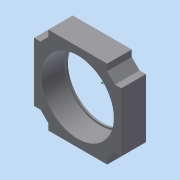
# Autodesk Inventor part: 20_Lens_holder_DIA_50mm
Saved by Autodesk Inventor 2019.4 (Build 234330000, 330)
## iProperties
Created: 2019-10-23
Part Number: 20_Lens_holder_DIA_50mm
Material: Generic
Document SubType Name: Modeling
Designer: marsikovabarbora
Density: 1 g/cm^3
Appearance: Default
Lens_diameter: 25,400 mm
Author: marsikovabarbora
Autodesk Inventor part; units mm, degrees
ref_plane "YZ Plane" through (0, 0, 0) normal (1, 0, 0) x (0, 1, 0)
ref_plane "XZ Plane" through (0, 0, 0) normal (0, 1, 0) x (-1, 0, 0)
ref_plane "XY Plane" through (0, 0, 0) normal (0, 0, 1) x (1, 0, 0)
sketch "Sketch1" plane through (0, 0, 0) normal (0, 0, 1) x (1, 0, 0)
  line L0 (-34.8609, 0) -> (34.8609, 0) construction
  line L1 (0, -34.8609) -> (0, 34.8609) construction
  line L2 (0, 0) -> (13.4339, 13.4339) construction
  line L3 (0, 0) -> (18.9985, 0) construction
  line L4 (0, 24.9006) -> (16.8, 24.9006)
  line L5 (16.8, 24.9006) -> (16.8, 21.2406)
  line L6 (16.8, 21.2406) -> (19.0203, 19.0203)
  line L7 (24.9006, 0) -> (24.9006, 16.8)
  line L8 (24.9006, 16.8) -> (21.2406, 16.8)
  line L9 (21.2406, 16.8) -> (19.0203, 19.0203)
  line L10 (0, 0) -> (-13.4339, 13.4339) construction
  line L11 (0, 0) -> (-18.9985, 0) construction
  line L12 (0, 24.9006) -> (-16.8, 24.9006)
  line L13 (-16.8, 24.9006) -> (-16.8, 21.2406)
  line L14 (-16.8, 21.2406) -> (-19.0203, 19.0203)
  line L15 (-24.9006, 0) -> (-24.9006, 16.8)
  line L16 (-24.9006, 16.8) -> (-21.2406, 16.8)
  line L17 (-21.2406, 16.8) -> (-19.0203, 19.0203)
  line L18 (0, 0) -> (13.4339, -13.4339) construction
  line L19 (0, -24.9006) -> (16.8, -24.9006)
  line L20 (16.8, -24.9006) -> (16.8, -21.2406)
  line L21 (16.8, -21.2406) -> (19.0203, -19.0203)
  line L22 (24.9006, 0) -> (24.9006, -16.8)
  line L23 (24.9006, -16.8) -> (21.2406, -16.8)
  line L24 (21.2406, -16.8) -> (19.0203, -19.0203)
  line L25 (0, 0) -> (-13.4339, -13.4339) construction
  line L26 (0, -24.9006) -> (-16.8, -24.9006)
  line L27 (-16.8, -24.9006) -> (-16.8, -21.2406)
  line L28 (-16.8, -21.2406) -> (-19.0203, -19.0203)
  line L29 (-24.9006, 0) -> (-24.9006, -16.8)
  line L30 (-24.9006, -16.8) -> (-21.2406, -16.8)
  line L31 (-21.2406, -16.8) -> (-19.0203, -19.0203)
  dimension "d0" = 45
  dimension "d1" = 3.14
  dimension "d2" = 3.66
  dimension "d3" = 16.8
  constraints: 60 end point, 24 symmetric about line, 5 point on line, 2 horizontal, 2 perpendicular, 1 equal length
  measures "d0" angle of L3 L2
  measures "d1" distance of L5.end L6.end
  measures "d2" distance of L4.end L5.end
  measures "d3" distance of L4.start L4.end
extrude "Thickness" add sketch "Sketch1" along normal blind 14
hole "Hole1" at (0, 0, 0) direction (0, 0, 1) diameter 41.2 end through all
sketch "Sketch2" plane through (0, 0, 0) normal (0, 0, -1) x (-1, 0, 0)
  circle A0 centre (0, 0) radius 20.6 projected
  line L0 (16.8, 24.9006) -> (-16.8, 24.9006) projected
  line L1 (-16.8, 24.9006) -> (-16.8, 21.2406) projected
  line L2 (-16.8, 21.2406) -> (-21.2406, 16.8) projected
  line L3 (-21.2406, 16.8) -> (-24.9006, 16.8) projected
  line L4 (-24.9006, 16.8) -> (-24.9006, -16.8) projected
  line L5 (-24.9006, -16.8) -> (-21.2406, -16.8) projected
  line L6 (-21.2406, -16.8) -> (-16.8, -21.2406) projected
  line L7 (-16.8, -21.2406) -> (-16.8, -24.9006) projected
  line L8 (-16.8, -24.9006) -> (16.8, -24.9006) projected
  line L9 (16.8, -24.9006) -> (16.8, -21.2406) projected
  line L10 (16.8, -21.2406) -> (21.2406, -16.8) projected
  line L11 (21.2406, -16.8) -> (24.9006, -16.8) projected
  line L12 (24.9006, -16.8) -> (24.9006, 16.8) projected
  line L13 (24.9006, 16.8) -> (21.2406, 16.8) projected
  line L14 (21.2406, 16.8) -> (16.8, 21.2406) projected
  line L15 (16.8, 21.2406) -> (16.8, 24.9006) projected
  circle A1 centre (0, 0) radius 19.6
  dimension "d17" = 1
  constraints: 1 centre point
  measures "d17" radial gap between concentric circles of A0 A1
extrude "Extrusion2" add sketch "Sketch2" against normal blind 1 contours A0
sketch "Sketch3" plane through (0, 0, 0) normal (0, 0, -1) x (-1, 0, 0)
  circle A0 centre (0, 0) radius 20.6 projected
  line L0 (-16.8, 24.9006) -> (16.8, 24.9006) projected
  line L1 (16.8, 24.9006) -> (16.8, 21.2406) projected
  line L2 (16.8, 21.2406) -> (21.2406, 16.8) projected
  line L3 (21.2406, 16.8) -> (24.9006, 16.8) projected
  line L4 (24.9006, 16.8) -> (24.9006, -16.8) projected
  line L5 (24.9006, -16.8) -> (21.2406, -16.8) projected
  line L6 (21.2406, -16.8) -> (16.8, -21.2406) projected
  line L7 (16.8, -21.2406) -> (16.8, -24.9006) projected
  line L8 (16.8, -24.9006) -> (-16.8, -24.9006) projected
  line L9 (-16.8, -24.9006) -> (-16.8, -21.2406) projected
  line L10 (-16.8, -21.2406) -> (-21.2406, -16.8) projected
  line L11 (-21.2406, -16.8) -> (-24.9006, -16.8) projected
  line L12 (-24.9006, -16.8) -> (-24.9006, 16.8) projected
  line L13 (-24.9006, 16.8) -> (-21.2406, 16.8) projected
  line L14 (-21.2406, 16.8) -> (-16.8, 21.2406) projected
  line L15 (-16.8, 21.2406) -> (-16.8, 24.9006) projected
  line L16 (16.8994, 25) -> (-16.8994, 25)
  line L17 (-16.8994, 25) -> (-16.8994, 21.2818)
  line L18 (-16.8994, 21.2818) -> (-21.2818, 16.8994)
  line L19 (-21.2818, 16.8994) -> (-25, 16.8994)
  line L20 (-25, 16.8994) -> (-25, -16.8994)
  line L21 (-25, -16.8994) -> (-21.2818, -16.8994)
  line L22 (-21.2818, -16.8994) -> (-16.8994, -21.2818)
  line L23 (-16.8994, -21.2818) -> (-16.8994, -25)
  line L24 (-16.8994, -25) -> (16.8994, -25)
  line L25 (16.8994, -25) -> (16.8994, -21.2818)
  line L26 (16.8994, -21.2818) -> (21.2818, -16.8994)
  line L27 (21.2818, -16.8994) -> (25, -16.8994)
  line L28 (25, -16.8994) -> (25, 16.8994)
  line L29 (25, 16.8994) -> (21.2818, 16.8994)
  line L30 (21.2818, 16.8994) -> (16.8994, 21.2818)
  line L31 (16.8994, 21.2818) -> (16.8994, 25)
  dimension "d22" = 50
  constraints: 32 end point, 15 other
  measures "d22" distance between parallel lines of L20 L28
extrude "Extrusion3" add sketch "Sketch3" against normal up to surface (14 mm away) contours L31 L30 L29 L28 L27 L26 L25 L24 L23 L22 L21 L20 L19 L18 L17 L16
equation "\"Lens_diameter\" = 25.4"
body "Solid1"
